Autodesk Inventor part; units mm, degrees
(part 2 of 2)
  line L921 (3.0068, -2.0174) -> (2.9345, -1.9555)
  line L922 (2.9345, -1.9555) -> (2.8626, -1.903)
  line L923 (2.8626, -1.903) -> (2.7917, -1.8599)
  line L924 (2.7917, -1.8599) -> (2.7225, -1.8259)
  line L925 (2.7225, -1.8259) -> (2.6555, -1.8008)
  line L926 (2.6555, -1.8008) -> (2.5915, -1.7843)
  line L927 (2.5915, -1.7843) -> (2.531, -1.7763)
  line L928 (2.531, -1.7763) -> (2.4747, -1.7762)
  line L929 (2.4747, -1.7762) -> (2.4229, -1.7838)
  line L930 (2.4229, -1.7838) -> (2.3764, -1.7986)
  line L931 (2.3764, -1.7986) -> (2.3356, -1.8202)
  line L932 (2.3356, -1.8202) -> (2.2971, -1.8521)
  line L933 (2.2971, -1.8521) -> (2.1557, -2.0138)
  line L934 (2.1557, -2.0138) -> (2.0859, -2.086)
  line L935 (2.0859, -2.086) -> (2.0136, -2.1559)
  line L936 (2.0136, -2.1559) -> (1.8519, -2.2972)
  line L937 (1.8519, -2.2972) -> (1.82, -2.3358)
  line L938 (1.82, -2.3358) -> (1.7984, -2.3766)
  line L939 (1.7984, -2.3766) -> (1.7836, -2.4231)
  line L940 (1.7836, -2.4231) -> (1.776, -2.4748)
  line L941 (1.776, -2.4748) -> (1.7761, -2.5312)
  line L942 (1.7761, -2.5312) -> (1.7842, -2.5917)
  line L943 (1.7842, -2.5917) -> (1.8006, -2.6557)
  line L944 (1.8006, -2.6557) -> (1.8257, -2.7226)
  line L945 (1.8257, -2.7226) -> (1.8597, -2.7919)
  line L946 (1.8597, -2.7919) -> (1.9028, -2.8628)
  line L947 (1.9028, -2.8628) -> (1.9553, -2.9347)
  line L948 (1.9553, -2.9347) -> (2.0173, -3.007)
  line L949 (2.0173, -3.007) -> (2.0888, -3.0789)
  line L950 (2.0888, -3.0789) -> (2.16, -3.1417)
  line L951 (2.16, -3.1417) -> (2.1859, -3.2049)
  line L952 (2.1859, -3.2049) -> (2.2134, -3.292)
  line L953 (2.2134, -3.292) -> (2.2401, -3.41)
  line L954 (2.2401, -3.41) -> (2.2601, -3.5527)
  line L955 (2.2601, -3.5527) -> (2.2666, -3.6359)
  line L956 (2.2666, -3.6359) -> (2.2698, -3.7256)
  line L957 (2.2698, -3.7256) -> (2.2692, -3.8217)
  line L958 (2.2692, -3.8217) -> (2.2643, -3.9235)
  line L959 (2.2643, -3.9235) -> (2.2544, -4.0331)
  line L960 (2.2544, -4.0331) -> (2.2392, -4.1474)
  line L961 (2.2392, -4.1474) -> (2.2179, -4.2687)
  line L962 (2.2179, -4.2687) -> (2.1904, -4.3944)
  line L963 (2.1904, -4.3944) -> (2.1602, -4.5092)
  arc A17 (1.6607, -4.7161) -> (2.1602, -4.5092) centre (-0.0001, 0) ccw
  line L964 (1.6607, -4.7161) -> (1.5582, -4.6562)
  line L965 (1.5582, -4.6562) -> (1.4499, -4.5868)
  line L966 (1.4499, -4.5868) -> (1.3491, -4.5161)
  line L967 (1.3491, -4.5161) -> (1.2575, -4.446)
  line L968 (1.2575, -4.446) -> (1.173, -4.3755)
  line L969 (1.173, -4.3755) -> (1.0975, -4.307)
  line L970 (1.0975, -4.307) -> (1.0292, -4.2395)
  line L971 (1.0292, -4.2395) -> (0.968, -4.1738)
  line L972 (0.968, -4.1738) -> (0.9138, -4.1104)
  line L973 (0.9138, -4.1104) -> (0.827, -3.9954)
  line L974 (0.827, -3.9954) -> (0.7624, -3.893)
  line L975 (0.7624, -3.893) -> (0.7203, -3.812)
  line L976 (0.7203, -3.812) -> (0.6939, -3.749)
  line L977 (0.6939, -3.749) -> (0.6999, -3.6542)
  line L978 (0.6999, -3.6542) -> (0.6996, -3.5528)
  line L979 (0.6996, -3.5528) -> (0.6923, -3.4579)
  line L980 (0.6923, -3.4579) -> (0.6785, -3.3699)
  line L981 (0.6785, -3.3699) -> (0.6589, -3.2893)
  line L982 (0.6589, -3.2893) -> (0.634, -3.2163)
  line L983 (0.634, -3.2163) -> (0.6044, -3.1512)
  line L984 (0.6044, -3.1512) -> (0.5708, -3.0943)
  line L985 (0.5708, -3.0943) -> (0.5337, -3.0458)
  line L986 (0.5337, -3.0458) -> (0.4939, -3.0059)
  line L987 (0.4939, -3.0059) -> (0.452, -2.9747)
  line L988 (0.452, -2.9747) -> (0.4086, -2.9523)
  line L989 (0.4086, -2.9523) -> (0.3644, -2.9387)
  line L990 (0.3644, -2.9387) -> (0.3146, -2.934)
  line L991 (0.3146, -2.934) -> (0.1004, -2.9484)
  line L992 (0.1004, -2.9484) -> (-0.0001, -2.9501)
  line L993 (-0.0001, -2.9501) -> (-0.1006, -2.9484)
  line L994 (-0.1006, -2.9484) -> (-0.3149, -2.934)
  line L995 (-0.3149, -2.934) -> (-0.3647, -2.9387)
  line L996 (-0.3647, -2.9387) -> (-0.4088, -2.9523)
  line L997 (-0.4088, -2.9523) -> (-0.4522, -2.9747)
  line L998 (-0.4522, -2.9747) -> (-0.4941, -3.0059)
  line L999 (-0.4941, -3.0059) -> (-0.534, -3.0458)
  line L1000 (-0.534, -3.0458) -> (-0.571, -3.0943)
  line L1001 (-0.571, -3.0943) -> (-0.6046, -3.1512)
  line L1002 (-0.6046, -3.1512) -> (-0.6342, -3.2163)
  line L1003 (-0.6342, -3.2163) -> (-0.6591, -3.2893)
  line L1004 (-0.6591, -3.2893) -> (-0.6788, -3.3699)
  line L1005 (-0.6788, -3.3699) -> (-0.6925, -3.4579)
  line L1006 (-0.6925, -3.4579) -> (-0.6998, -3.5528)
  line L1007 (-0.6998, -3.5528) -> (-0.7001, -3.6542)
  line L1008 (-0.7001, -3.6542) -> (-0.6941, -3.749)
  line L1009 (-0.6941, -3.749) -> (-0.7205, -3.812)
  line L1010 (-0.7205, -3.812) -> (-0.7627, -3.893)
  line L1011 (-0.7627, -3.893) -> (-0.8272, -3.9954)
  line L1012 (-0.8272, -3.9954) -> (-0.914, -4.1104)
  line L1013 (-0.914, -4.1104) -> (-0.9682, -4.1738)
  line L1014 (-0.9682, -4.1738) -> (-1.0294, -4.2395)
  line L1015 (-1.0294, -4.2395) -> (-1.0978, -4.307)
  line L1016 (-1.0978, -4.307) -> (-1.1732, -4.3755)
  line L1017 (-1.1732, -4.3755) -> (-1.2577, -4.446)
  line L1018 (-1.2577, -4.446) -> (-1.3493, -4.5161)
  line L1019 (-1.3493, -4.5161) -> (-1.4501, -4.5868)
  line L1020 (-1.4501, -4.5868) -> (-1.5584, -4.6562)
  line L1021 (-1.5584, -4.6562) -> (-1.661, -4.7161)
  arc A18 (-2.1605, -4.5092) -> (-1.661, -4.7161) centre (-0.0001, 0) ccw
  line L1022 (-2.1605, -4.5092) -> (-2.1906, -4.3944)
  line L1023 (-3.3452, 2.6801) -> (-3.6666, 2.5292)
  line L1024 (-3.6666, 2.5292) -> (-3.9743, 2.3925)
  line L1025 (-3.9743, 2.3925) -> (-4.2682, 2.2692)
  line L1026 (-4.2682, 2.2692) -> (-4.5472, 2.1589)
  line L1027 (-4.5472, 2.1589) -> (-4.8121, 2.0607)
  line L1028 (-4.8121, 2.0607) -> (-5.0226, 1.9866)
  line L1029 (-5.0226, 1.9866) -> (-5.0656, 1.9647)
  line L1030 (-5.0656, 1.9647) -> (-5.0795, 1.9535)
  line L1031 (-5.0795, 1.9535) -> (-5.0884, 1.9423)
  line L1032 (-5.0884, 1.9423) -> (-5.0922, 1.9312)
  line L1033 (-5.0922, 1.9312) -> (-5.0901, 1.8783)
  line L1034 (-5.0901, 1.8783) -> (-5.0769, 1.5338)
  line L1035 (-5.0769, 1.5338) -> (-5.0661, 1.1891)
  line L1036 (-5.0661, 1.1891) -> (-5.0645, 1.1362)
  line L1037 (-5.0645, 1.1362) -> (-5.0599, 1.1254)
  line L1038 (-5.0599, 1.1254) -> (-5.0502, 1.1148)
  line L1039 (-5.0502, 1.1148) -> (-5.0356, 1.1046)
  line L1040 (-5.0356, 1.1046) -> (-4.9911, 1.0858)
  line L1041 (-4.9911, 1.0858) -> (-4.776, 1.0266)
  line L1042 (-4.776, 1.0266) -> (-4.5049, 0.947)
  line L1043 (-4.5049, 0.947) -> (-4.2189, 0.8566)
  line L1044 (-4.2189, 0.8566) -> (-3.917, 0.7541)
  line L1045 (-3.917, 0.7541) -> (-3.6006, 0.6392)
  line L1046 (-3.6006, 0.6392) -> (-3.2695, 0.511)
  line L1047 (-3.2695, 0.511) -> (-3.0019, 0.4017)
  arc A19 (-3.0019, -0.4018) -> (-3.0019, 0.4017) centre (-49.0001, -0.0001) ccw
  line L1048 (-3.0019, -0.4018) -> (-3.2695, -0.5112)
  line L1049 (-3.2695, -0.5112) -> (-3.6006, -0.6393)
  line L1050 (-3.6006, -0.6393) -> (-3.917, -0.7542)
  line L1051 (-3.917, -0.7542) -> (-4.2189, -0.8567)
  line L1052 (-4.2189, -0.8567) -> (-4.5049, -0.9472)
  line L1053 (-4.5049, -0.9472) -> (-4.776, -1.0268)
  line L1054 (-4.776, -1.0268) -> (-4.9911, -1.086)
  line L1055 (-4.9911, -1.086) -> (-5.0356, -1.1048)
  line L1056 (-5.0356, -1.1048) -> (-5.0502, -1.115)
  line L1057 (-5.0502, -1.115) -> (-5.0599, -1.1255)
  line L1058 (-5.0599, -1.1255) -> (-5.0645, -1.1364)
  line L1059 (-5.0645, -1.1364) -> (-5.0661, -1.1893)
  line L1060 (-5.0661, -1.1893) -> (-5.0769, -1.5339)
  line L1061 (-5.0769, -1.5339) -> (-5.0901, -1.8785)
  line L1062 (-5.0901, -1.8785) -> (-5.0922, -1.9313)
  line L1063 (-5.0922, -1.9313) -> (-5.0884, -1.9425)
  line L1064 (-5.0884, -1.9425) -> (-5.0795, -1.9537)
  line L1065 (-5.0795, -1.9537) -> (-5.0656, -1.9649)
  line L1066 (-5.0656, -1.9649) -> (-5.0226, -1.9868)
  line L1067 (-5.0226, -1.9868) -> (-4.8121, -2.0608)
  line L1068 (-4.8121, -2.0608) -> (-4.5472, -2.1591)
  line L1069 (-4.5472, -2.1591) -> (-4.2682, -2.2693)
  line L1070 (-4.2682, -2.2693) -> (-3.9743, -2.3926)
  line L1071 (-3.9743, -2.3926) -> (-3.6666, -2.5293)
  line L1072 (-3.6666, -2.5293) -> (-3.3452, -2.6802)
  line L1073 (-3.3452, -2.6802) -> (-3.0859, -2.808)
  arc A20 (-3.1419, -3.6095) -> (-3.0859, -2.808) centre (-49.0001, -0.0001) ccw
  line L1074 (-3.1419, -3.6095) -> (-3.4165, -3.7)
  line L1075 (-3.4165, -3.7) -> (-3.7558, -3.8047)
  line L1076 (-3.7558, -3.8047) -> (-4.0795, -3.8972)
  line L1077 (-4.0795, -3.8972) -> (-4.3877, -3.9784)
  line L1078 (-4.3877, -3.9784) -> (-4.6793, -4.0487)
  line L1079 (-4.6793, -4.0487) -> (-4.9553, -4.1092)
  line L1080 (-4.9553, -4.1092) -> (-5.1741, -4.1532)
  line L1081 (-5.1741, -4.1532) -> (-5.2197, -4.1689)
  line L1082 (-5.2197, -4.1689) -> (-5.2351, -4.178)
  line L1083 (-5.2351, -4.178) -> (-5.2454, -4.1879)
  line L1084 (-5.2454, -4.1879) -> (-5.2508, -4.1984)
  line L1085 (-5.2508, -4.1984) -> (-5.256, -4.2511)
  line L1086 (-5.256, -4.2511) -> (-5.2909, -4.5941)
  line L1087 (-5.2909, -4.5941) -> (-5.3281, -4.9369)
  line L1088 (-5.3281, -4.9369) -> (-5.3339, -4.9895)
  line L1089 (-5.3339, -4.9895) -> (-5.3309, -5.0009)
  line L1090 (-5.3309, -5.0009) -> (-5.3228, -5.0127)
  line L1091 (-5.3228, -5.0127) -> (-5.3097, -5.0248)
  line L1092 (-5.3097, -5.0248) -> (-5.2683, -5.0496)
  line L1093 (-5.2683, -5.0496) -> (-5.0635, -5.1382)
  line L1094 (-5.0635, -5.1382) -> (-4.8061, -5.2547)
  line L1095 (-4.8061, -5.2547) -> (-4.5355, -5.3841)
  line L1096 (-4.8061, 5.2546) -> (-5.0635, 5.138)
  line L1097 (-5.0635, 5.138) -> (-5.2683, 5.0495)
  line L1098 (-5.2683, 5.0495) -> (-5.3097, 5.0247)
  line L1099 (-5.3097, 5.0247) -> (-5.3228, 5.0125)
  line L1100 (-5.3228, 5.0125) -> (-5.3309, 5.0007)
  line L1101 (-5.3309, 5.0007) -> (-5.3339, 4.9893)
  line L1102 (-5.3339, 4.9893) -> (-5.3281, 4.9367)
  line L1103 (-5.3281, 4.9367) -> (-5.2909, 4.5939)
  line L1104 (-5.2909, 4.5939) -> (-5.256, 4.2509)
  line L1105 (-5.256, 4.2509) -> (-5.2508, 4.1982)
  line L1106 (-5.2508, 4.1982) -> (-5.2454, 4.1878)
  line L1107 (-5.2454, 4.1878) -> (-5.2351, 4.1779)
  line L1108 (-5.2351, 4.1779) -> (-5.2197, 4.1687)
  line L1109 (-5.2197, 4.1687) -> (-5.1741, 4.1531)
  line L1110 (-5.1741, 4.1531) -> (-4.9553, 4.109)
  line L1111 (-4.9553, 4.109) -> (-4.6793, 4.0486)
  line L1112 (-4.6793, 4.0486) -> (-4.3877, 3.9783)
  line L1113 (-4.3877, 3.9783) -> (-4.0795, 3.8971)
  line L1114 (-4.0795, 3.8971) -> (-3.7558, 3.8045)
  line L1115 (-3.7558, 3.8045) -> (-3.4165, 3.6998)
  line L1116 (-3.4165, 3.6998) -> (-3.1419, 3.6094)
  arc A21 (-3.0859, 2.8078) -> (-3.1419, 3.6094) centre (-49.0001, -0.0001) ccw
  line L1117 (-3.0859, 2.8078) -> (-3.3452, 2.6801)
  point P0 (-2.1605, -4.5092)
  point P1 (-1.661, -4.7161)
  point P2 (1.6607, -4.7161)
  point P3 (2.1602, -4.5092)
  point P4 (4.509, -2.1604)
  point P5 (4.7159, -1.6609)
  point P6 (4.7159, 1.6608)
  point P7 (4.509, 2.1603)
  point P8 (2.1602, 4.5091)
  point P9 (1.6607, 4.716)
  point P10 (-1.661, 4.716)
  point P11 (-2.1605, 4.5091)
  point P12 (-4.5093, 2.1603)
  point P13 (-4.7162, 1.6608)
  point P14 (-4.7162, -1.6609)
  point P15 (-4.5093, -2.1604)
  constraints: 2236 end point, 44 point on circle, 22 centre point
extrude "Extrusion5" add sketch "Sketch5" along normal blind 8 from surface at 0 contours L0 L1 L2 L3 L4 L5 L6 L7 L8 L9 L10 L11 L12 L13 L14 L15 L16 L17 L18 L19 L20 L21 L22 L23 L24 L25 L26 L27 L28 L29 L30 L31 L32 L33 L34 L35 L36 L37 L38 L39 L40 L41 L42 L43 L44 L45 L46 L47 L48 L49 L50 L51 L52 L53 L54 L55 L56 A0 L57 L58 L59 L60 L61 L62 L63 L64 L65 L66 L67 L68 L69 L70 L71 L72 L73 L74 L75 L76 L77 L78 L79 L80 L81 L82 L83 L84 L85 L86 L87 L88 L89 L90 L91 L92 L93 L94 L95 L96 L97 L98 L99 L100 L101 L102 L103 L104 L105 L106 L107 L108 L109 L110 L111 L112 L113 L114 A1 L115 L116 L117 L118 L119 L120 L121 L122 L123 L124 L125 L126 L127 L128 L129 L130 L131 L132 L133 L134 L135 L136 L137 L138 L139 L140 L141 L142 L143 L144 L145 L146 L147 L148 L149 L150 L151 L152 L153 L154 L155 L156 L157 L158 L159 L160 L161 L162 L163 L164 L165 L166 L167 L168 L169 L170 L171 L172 A2 L173 L174 L175 L176 L177 L178 L179 L180 L181 L182 L183 L184 L185 L186 L187 L188 L189 L190 L191 L192 L193 L194 L195 L196 L197 L198 L199 L200 L201 L202 L203 L204 L205 L206 L207 L208 L209 L210 L211 L212 L213 L214 L215 L216 L217 L218 L219 L220 L221 L222 L223 L224 L225 L226 L227 L228 L229 L230 A3 L231 L232 L233 L234 L235 L236 L237 L238 L239 L240 L241 L242 L243 L244 L245 L246 L247 L248 L249 L250 L251 L252 L253 L254 L255 L256 L257 L258 L259 L260 L261 L262 L263 L264 L265 L266 L267 L268 L269 L270 L271 L272 L273 L274 L275 L276 L277 L278 L279 L280 L281 L282 L283 L284 L285 L286 L287 L288 A4 L289 L290 L291 L292 L293 L294 L295 L296 L297 L298 L299 L300 L301 L302 L303 L304 L305 L306 L307 L308 L309 L310 L311 L312 L313 L314 L315 L316 L317 L318 L319 L320 L321 L322 L323 L324 L325 L326 L327 L328 L329 L330 L331 L332 L333 L334 L335 L336 L337 L338 L339 L340 L341 L342 L343 L344 L345 L346 A5 L347 L348 L349 L350 L351 L352 L353 L354 L355 L356 L357 L358 L359 L360 L361 L362 L363 L364 L365 L366 L367 L368 L369 L370 L371 L372 L373 L374 L375 L376 L377 L378 L379 L380 L381 L382 L383 L384 L385 L386 L387 L388 L389 L390 L391 L392 L393 L394 L395 L396 L397 L398 L399 L400 L401 L402 L403 L404 A6 L405 L406 L407 L408 L409 L410 L411 L412 L413 L414 L415 L416 L417 L418 L419 L420 L421 L422 L423 L424 L425 L426 L427 L428 L429 L430 L431 L432 L433 L434 L435 L436 L437 L438 L439 L440 L441 L442 L443 L444 L445 L446 L447 L448 L449 L450 L451 L452 L453 L454 L455 L456 L457 L458 L459 L460 L461 L462 A7 L463
sketch "Sketch2" plane through (0, 0, 3) normal (0, 0, 1) x (1, 0, 0)
  circle A0 centre (-6.35, 0) radius 1.6
  point P0 (0, 0)
  dimension "d4" = 3.2
  dimension "d5" = 6.35
  constraints: 1 centre point
  measures "d4" diameter of A0
  measures "d5" distance of point (0, 0) A0.centre
extrude "Extrusion2" cut sketch "Sketch2" along normal mid plane 50
pattern_circular "Circular Pattern1" count 4 over 360 about axis through (0, 0, 0) along (0, 0, 1) of "Extrusion2"
sketch "Sketch8" plane through (0, 0, 3) normal (0, 0, 1) x (1, 0, 0)
  circle A0 centre (0, 6.35) radius 3
  arc A1 (-1.6, 8.8877) -> (1.6, 8.8877) centre (0, 6.35) ccw
  line L0 (-1.6, 8.8877) -> (-1.6, 11.8929)
  circle A2 centre (0, 0) radius 12 projected
  line L1 (1.6, 8.8877) -> (1.6, 11.8929)
  arc A3 (1.6, 11.8929) -> (-1.6, 11.8929) centre (0, 0) ccw
  circle A4 centre (0, 6.35) radius 1.6 projected
  dimension "d29" = 6
  dimension "d30" = 1.6
  dimension "d31" = 1.6
  constraints: 6 point on circle, 4 end point, 2 centre point, 2 coincident, 2 vertical, 1 concentric, 4 other
  measures "d30" distance from line of L1 A1.centre
  measures "d31" distance from line of A1.centre L0
extrude "Extrusion7" cut sketch "Sketch8" along normal blind 8 contours A0 | A0 L0 A2 L1 | A4 picked at (0.8239, 11.0707)
sketch "Sketch9" plane through (0, 0, 11) normal (0, 0, -1) x (-1, 0, 0)
  arc A0 (-3, 6.35) -> (3, 6.35) centre (0, 6.35) ccw
  line L0 (3, 6.35) -> (3, 11.619)
  arc A1 (-1.6, 11.8929) -> (1.6, 11.8929) centre (0, 0) ccw projected
  line L1 (-3, 6.35) -> (-3, 11.619)
  arc A2 (3, 11.619) -> (-3.3238, 11.5305) centre (0, 0) ccw
  circle A3 centre (0, 6.35) radius 1.6 projected
  point P0 (1.6, 11.8929)
  dimension "d28" = 3
  constraints: 7 point on circle, 4 end point, 2 centre point, 2 concentric, 2 tangent, 1 coincident, 1 parallel, 1 vertical
  measures "d28" radius of A0
extrude "Extrusion8" cut sketch "Sketch9" against normal blind 3.5 contours L1 A1 A2 L0 A0 | A3
pattern_circular "Circular Pattern3" count 4 over 360 about axis through (0, 0, 0) along (0, 0, 1) of "Extrusion7", "Extrusion8"
sketch "Sketch10" plane through (0, 0, 3) normal (0, 0, -1) x (-1, 0, 0)
  circle A0 centre (0, 0) radius 2.6
  circle A1 centre (0, 0) radius 2.6 projected
  constraints: 1 centre point, 1 coincident, 1 concentric
extrude "Extrusion9" cut sketch "Sketch10" against normal blind 12
body "Solid1"
